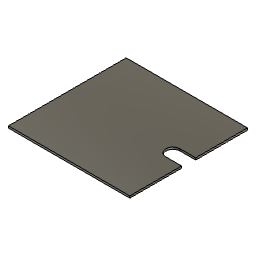
Floor  1 v8 (Autodesk Fusion 360 design; units mm, degrees)
Autodesk Fusion 360 part; units mm, degrees
note: some values were not read from the file. Set by a fixed rule: which sketch regions a step uses.
sketch "Sketch1" plane through (0, 0, 0) normal (0, 0, 1) x (1, 0, 0)
  line L0 (-154.5, 150) -> (154.5, 150)
  line L1 (154.5, -150) -> (-154.5, -150)
  line L2 (-154.5, -150) -> (-154.5, 150)
  line L3 (-154.5, 150) -> (154.5, -150) construction
  line L4 (154.5, 18) -> (114.5, 18)
  line L5 (114.5, -18) -> (154.5, -18)
  arc A0 (114.5, 18) -> (114.5, -18) centre (114.5, 0) ccw
  line L6 (154.5, 150) -> (154.5, 18)
  line L7 (154.5, -18) -> (154.5, -150)
  dimension "d1" = 309
  dimension "d2" = 300
  dimension "d6" = 36
  dimension "d7" = 40
  dimension "d8" = 150
  constraint horizontal L0
  constraint vertical L6
  constraint horizontal L1
  constraint vertical L2
  constraint midpoint origin L3
  constraint horizontal L4
  constraint horizontal L5
  constraint collinear L6 L7
  constraint tangent L4 A0
  constraint tangent L5 A0
  measures "d1" distance of L0.start L0.end
  measures "d2" distance of L0.start L1.end
  measures "d6" distance of L4.end L5.start
  measures "d7" distance of L4.start L4.end
  measures "d8" vertical distance of L0.end A0.centre
extrude "Extrude1" add sketch "Sketch1" along normal blind 5
